Autodesk Fusion 360 part; units mm, degrees
(part 2 of 2)
  point P201 (-276.3266, 286.1027)
  point P202 (-276.9844, 282.8707)
  point P203 (-276.9949, 277.0329)
  point P204 (-276.8525, 271.4361)
  point P205 (-276.6299, 264.3263)
  point P206 (-276.5848, 257.7924)
  point P207 (-276.4514, 250.895)
  point P208 (-276.1743, 242.9378)
  point P209 (-275.811, 234.3146)
  point P210 (-275.4044, 227.5665)
  point P211 (-274.6441, 219.485)
  point P212 (-274.0319, 211.8582)
  point P213 (-267.9751, 204.4177)
  point P214 (-267.5442, 204.0898)
  point P215 (-267.3032, 203.2903)
  point P216 (-267.3192, 200.9915)
  point P217 (-267.35, 196.5777)
  point P218 (-267.7146, 193.925)
  point P219 (-269.1647, 192.1255)
  point P220 (-270.7582, 191.5785)
  point P221 (-272.6815, 192.2515)
  point P222 (-273.9897, 193.8335)
  point P223 (-274.2623, 195.9663)
  point P224 (-274.277, 201.1247)
  point P225 (-274.5808, 203.6298)
  point P226 (-274.5418, 204.3737)
  point P227 (-274.1861, 204.4557)
  point P228 (-215.7268, 203.2532)
  point P229 (-215.9928, 201.7068)
  point P230 (-215.5506, 196.8036)
  point P231 (-214.5783, 192.288)
  dimension "d165" = 2.3535
  dimension "d166" = 2.2794
  constraint midpoint S15.end L0
  constraint midpoint S15.start L1
  constraint perpendicular L2 L3
  constraint coincident L2 L4.start
  constraint coincident L2 L5.end
  constraint perpendicular L2 L5
  measures "d165" distance of S12.start L2.start
  measures "d166" distance of S10.start L4.start
extrude "Extrude2" cut sketch "Sketch3" against normal blind 5
equation "d163 = 2.5 mm + 10 mm"
